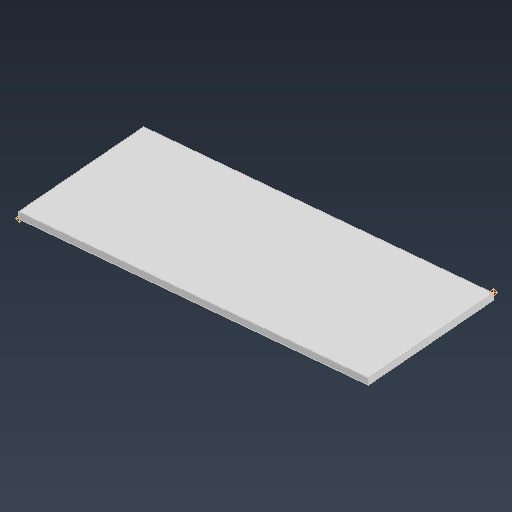
# Autodesk Inventor part: goalPanelBottomSlope
Saved by Autodesk Inventor 2021.4 (Build 254397000, 397)
## iProperties
Created: 2022-03-22
Part Number: goalPanelBottomSlope
Material: Generic
Document SubType Name: Modeling
Designer: jo_ki
Density: 1 g/cm^3
Appearance: Default
Author: jo_ki
Autodesk Inventor part; units mm, degrees
ref_plane "YZ Plane" through (0, 0, 0) normal (1, 0, 0) x (0, 1, 0)
derived "Mastersketch.ipt"
ref_plane "Work Plane3" through (0, 0, 0) normal (-0.7071068, 0, 0.7071068) x (0, 1, 0)
ref_plane "Work Plane1" through (0, 0, 0) normal (-0.1736482, 0.9848078, 0) x (0, 0, 1)
ref_plane "Work Plane2" through (0, 0, 0) normal (0, 0.9848078, 0.1736482) x (1, 0, 0)
ref_plane "Work Plane4" through (0, 0, 0) normal (0.0874861, -0.9923167, -0.0874861) x (-0.7071068, 0, -0.7071068)
sketch "Sketch1" plane through (0, 0, 0) normal (0.0874861, -0.9923167, -0.0874861) x (-0.7071068, 0, -0.7071068)
  line L0 (160.2104, -158.9795) -> (-160.2104, 158.9795) projected
  line L1 (160.2104, 158.9795) -> (-160.2104, -158.9795) projected
  line L2 (51.3476, -112.9399) -> (-113.3326, 50.475)
  line L3 (-113.3326, 50.475) -> (-51.3476, 112.9399)
  line L4 (-51.3476, 112.9399) -> (113.3326, -50.475)
  line L5 (113.3326, -50.475) -> (51.3476, -112.9399)
  line L6 (51.3476, -112.9399) -> (-51.3476, 112.9399) construction
  line L7 (-113.3326, 50.475) -> (113.3326, -50.475) construction
  point P0 (0, 0)
  dimension "d3" = 232
  dimension "d4" = 88
  constraints: 12 end point, 3 parallel, 2 midpoint, 1 perpendicular
  measures "d3" distance of L3.end L4.end
  measures "d4" distance of L2.end L3.end
extrude "Extrusion1" add sketch "Sketch1" along normal blind 4
sketch "Sketch2" plane through (0, 0, 0) normal (0, 1, 0) x (-1, 0, 0)
  line L0 (112, -40) -> (-112, -40)
  line L1 (-112, -40) -> (-112, 40)
  line L2 (-112, 40) -> (112, 40)
  line L3 (112, 40) -> (112, -40)
  line L4 (112, -40) -> (-112, 40) construction
  line L5 (-112, -40) -> (112, 40) construction
  point P0 (0, 0)
  dimension "d9" = 224
  dimension "d10" = 80
  constraints: 12 end point, 2 midpoint, 2 parallel, 1 horizontal, 1 perpendicular
  measures "d9" distance of L0.start L0.end
  measures "d10" distance of L0.end L1.end
extrude "Extrusion2" cut sketch "Sketch2" against normal through all both and the other way through all keep common part
equation "\"d7\" = goalPanel_thickness"
equation "\"goalPanel_thickness\" = 4"
body "Solid1"
